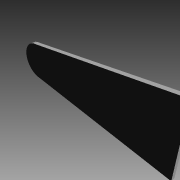
# Autodesk Inventor part: Headlight_Mounting_Bracket
Saved by Autodesk Inventor 2016 (Build 200138000, 138)
## iProperties
Created: 2015-08-10
Part Number: Headlight_Mounting_Bracket
Material: Generic
Document SubType Name: Modeling
Designer: Yann
Density: 1 g/cm^3
Appearance: Default
Author: Yann
Autodesk Inventor part; units mm, degrees
ref_plane "YZ Plane" through (0, 0, 0) normal (1, 0, 0) x (0, 1, 0)
ref_plane "XZ Plane" through (0, 0, 0) normal (0, 1, 0) x (-1, 0, 0)
ref_plane "XY Plane" through (0, 0, 0) normal (0, 0, 1) x (1, 0, 0)
sketch "Sketch1" plane through (0, 0, 0) normal (0, 1, 0) x (-1, 0, 0)
  line L0 (0, 12.655) -> (-92.4897, 24.1555)
  line L1 (-92.4897, 24.1555) -> (-92.4897, -24.1555)
  line L2 (-92.4897, -24.1555) -> (0, -12.655)
  arc A0 (0, -12.655) -> (0, 12.655) centre (0, 0) ccw
  line L3 (-113.5186, 0) -> (33.6839, 0) construction
  constraints: 6 end point, 2 point on circle, 1 centre point, 1 coincident, 1 vertical, 1 other
extrude "Extrusion1" add sketch "Sketch1" along normal blind 3
body "Solid1"
